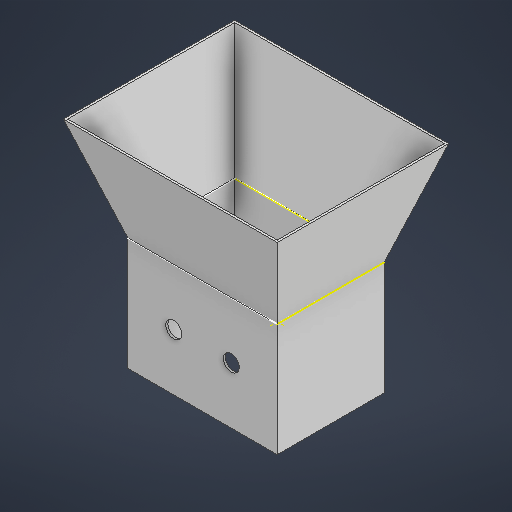
# Autodesk Inventor part: tolva
Saved by Autodesk Inventor 2026.1 (Build 301233020, 233B)
## iProperties
Created: 2025-11-30
Part Number: tolva
Material: Genérico
Document SubType Name: Modeling
Designer: TUF GAMING F15
Density: 1 g/cm^3
Appearance: Valor por defecto
Author: TUF GAMING F15
Autodesk Inventor part; units mm, degrees
ref_plane "YZ Plane" through (0, 0, 0) normal (1, 0, 0) x (0, 1, 0)
ref_plane "XZ Plane" through (0, 0, 0) normal (0, 1, 0) x (-1, 0, 0)
sketch "Boceto1" plane through (0, 0, 0) normal (0, 0, 1) x (1, 0, 0)
  circle A0 centre (0, 0) radius 62.5 construction
  circle A1 centre (0, 0) radius 20 construction
  line L0 (20, 0) -> (84, 0)
  circle A2 centre (84, 0) radius 62.5 construction
  circle A3 centre (84, 0) radius 20 construction
  line L1 (-62.5, 0) -> (-64, 0) construction
  line L2 (146.5, 0) -> (148, 0) construction
  line L3 (0, 62.5) -> (0, 82.5) construction
  line L4 (-64, 0) -> (-64, 82.5) construction
  line L5 (-64, 82.5) -> (0, 82.5)
  line L6 (0, 82.5) -> (148, 82.5)
  line L7 (148, 82.5) -> (148, 0) construction
  line L8 (-64, 0) -> (-64, -82.5) construction
  line L9 (-64, -82.5) -> (0, -82.5)
  line L10 (0, -82.5) -> (148, -82.5)
  line L11 (148, -82.5) -> (148, 0) construction
  line L12 (-64, 82.5) -> (-67, 82.5)
  line L13 (-67, 82.5) -> (-67, -82.5)
  line L14 (-67, -82.5) -> (-64, -82.5)
  line L15 (148, 82.5) -> (151, 82.5)
  line L16 (151, 82.5) -> (151, -82.5)
  line L17 (151, -82.5) -> (148, -82.5)
  circle A4 centre (0, 0) radius 12.7 construction
  line L18 (0, 12.7) -> (8.9803, 8.9803) construction
  line L19 (8.9803, 8.9803) -> (12.7, 0) construction
  line L20 (12.7, 0) -> (8.9803, -8.9803) construction
  line L21 (8.9803, -8.9803) -> (0, -12.7) construction
  line L22 (0, -12.7) -> (-8.9803, -8.9803) construction
  line L23 (-8.9803, -8.9803) -> (-12.7, 0) construction
  line L24 (-12.7, 0) -> (-8.9803, 8.9803) construction
  line L25 (-8.9803, 8.9803) -> (0, 12.7) construction
  circle A5 centre (0, 0) radius 11.7333
  circle A6 centre (84, 0) radius 12.7 construction
  line L26 (84, 12.7) -> (92.9803, 8.9803) construction
  line L27 (92.9803, 8.9803) -> (96.7, 0) construction
  line L28 (96.7, 0) -> (92.9803, -8.9803) construction
  line L29 (92.9803, -8.9803) -> (84, -12.7) construction
  line L30 (84, -12.7) -> (75.0197, -8.9803) construction
  line L31 (75.0197, -8.9803) -> (71.3, 0) construction
  line L32 (71.3, 0) -> (75.0197, 8.9803) construction
  line L33 (75.0197, 8.9803) -> (84, 12.7) construction
  circle A7 centre (84, 0) radius 11.7333
  dimension "d1" = 40
  dimension "d3" = 125
  dimension "d35" = 25.4
  dimension "d36" = 25.4
  dimension "d0" = 125
  dimension "d2" = 64
  dimension "d4" = 40
  dimension "d5" = 1.5
  dimension "d6" = 1.5
  dimension "d7" = 20
  dimension "d8" = 3
  dimension "d9" = 3
  constraints: 68 end point, 11 coincident, 6 perpendicular, 5 horizontal, 4 centre point, 3 symmetric about line, 2 horizontal alignment, 2 point on circle, 2 point on line, 2 vertical, 2 vertical alignment, 42 other
  measures "d0" diameter of A0
  measures "d2" distance of L0.start L0.end
  measures "d4" diameter of A3
  measures "d5" distance of L1.start L1.end
  measures "d6" distance of L2.start L2.end
  measures "d7" distance of L3.start L3.end
  measures "d8" distance of L4.end L12.end
  measures "d9" distance of L6.end L15.end
extrude "Extrusión1" add sketch "Boceto1" along normal blind 3
sketch "Boceto2" plane through (0, 0, 3) normal (0, 0, 1) x (1, 0, 0)
  line L0 (151, 82.5) -> (-67, 82.5) projected
  line L1 (-67, 82.5) -> (-64, 82.5)
  line L2 (-64, 82.5) -> (-64, -82.5)
  line L3 (-67, -82.5) -> (151, -82.5) projected
  line L4 (-67, 82.5) -> (-67, -82.5)
  line L5 (-64, -82.5) -> (-67, -82.5)
  line L6 (151, 82.5) -> (148, 82.5)
  line L7 (148, 82.5) -> (148, -82.5)
  line L8 (151, -82.5) -> (151, 82.5) projected
  line L9 (148, -82.5) -> (151, -82.5)
  line L10 (151, -82.5) -> (151, 82.5)
  point P0 (0, 0)
  dimension "d12" = 3
  dimension "d13" = 3
  constraints: 16 end point, 4 point on line, 3 perpendicular, 1 collinear, 1 horizontal, 1 vertical
  measures "d12" distance of L0.end L1.end
  measures "d13" distance of L0.start L6.end
extrude "Extrusión2" add sketch "Boceto2" along normal blind 75 contours L8 L3 L7 L0 | L2 L3 L4 L0
mirror "Simetría1" about plane through (149.5, 0, 78) normal (0, 0, 1) of "Extrusión2", "Extrusión1"
ref_plane "Plano de trabajo1" through (-67, 232.5, 0) normal (0, 1, 0) x (1, 0, 0)
sketch "Boceto4" plane through (-67, 232.5, 0) normal (0, 1, 0) x (1, 0, 0)
  line L0 (215, -153) -> (3, -153) projected
  line L1 (3, -153) -> (3, -203) construction
  line L2 (3, -153) -> (-47, -153) construction
  line L3 (3, -153) -> (53, -153) construction
  line L4 (215, -3) -> (215, -153) projected
  line L5 (215, -3) -> (215, 47) construction
  line L6 (215, -3) -> (265, -3) construction
  line L7 (215, -3) -> (265, -3) construction
  line L8 (265, -3) -> (265, 47) construction
  line L9 (265, 47) -> (215, 47) construction
  line L10 (3, -203) -> (-47, -203) construction
  line L11 (-47, -203) -> (-47, -153) construction
  line L12 (-47, -203) -> (265, -203)
  line L13 (265, -203) -> (265, 47)
  line L14 (265, 47) -> (-47, 47)
  line L15 (-47, 47) -> (-47, -203)
  line L16 (-47, -203) -> (-47, -206) construction
  line L17 (-47, -203) -> (-50, -203) construction
  line L18 (-50, -203) -> (-50, -206) construction
  line L19 (-50, -206) -> (-47, -206) construction
  line L20 (265, 47) -> (268, 47) construction
  line L21 (265, 47) -> (265, 50) construction
  line L22 (265, 50) -> (268, 50) construction
  line L23 (268, 50) -> (268, 47) construction
  line L24 (-50, -206) -> (268, -206)
  line L25 (268, -206) -> (268, 50)
  line L26 (268, 50) -> (-50, 50)
  line L27 (-50, 50) -> (-50, -206)
  point P0 (67, 0)
  dimension "d18" = 50
  dimension "d20" = 50
  dimension "d21" = 180
  dimension "d22" = 50
  dimension "d24" = 50
  dimension "d25" = 0
  dimension "d26" = 3
  dimension "d27" = 3
  dimension "d28" = 3
  dimension "d29" = 3
  constraints: 52 end point, 10 perpendicular, 7 horizontal, 5 parallel, 4 vertical, 2 collinear
  measures "d18" distance of L0.end L1.end
  measures "d20" distance of L0.end L2.end
  measures "d21" angle of L2 L3
  measures "d22" distance of L4.start L5.end
  measures "d24" distance of L4.start L6.end
  measures "d25" distance between parallel lines of L6 L7
  measures "d26" distance of L10.end L16.end
  measures "d27" distance of L10.end L17.end
  measures "d28" distance of L8.end L20.end
  measures "d29" distance of L8.end L21.end
sketch "Boceto5" plane through (-67, 82.5, 0) normal (0, 1, 0) x (1, 0, 0)
  line L0 (218, 0) -> (0, 0) projected
  line L1 (218, 0) -> (218, -156) projected
  line L2 (0, 0) -> (218, 0)
  line L3 (218, 0) -> (218, -156)
  line L4 (218, -156) -> (0, -156)
  line L5 (0, -156) -> (0, 0)
  line L6 (215, -3) -> (3, -3) projected
  line L7 (3, -3) -> (215, -3)
  line L8 (215, -3) -> (215, -153)
  line L9 (215, -153) -> (3, -153)
  line L10 (3, -153) -> (3, -3)
  point P0 (67, 0)
  constraints: 16 end point, 4 parallel, 2 horizontal, 2 perpendicular
loft "Solevación1" add profiles "Boceto4" section 1 edges at (151, 82.5, 78) (42, 82.5, 0) (-67, 82.5, 78) (42, 82.5, 156) contours L15 L14 L13 L12
shell "Vaciado1" thickness 3 removed faces 2 at (94, 232.5, 119.6667) at (77.3333, 82.5, 103)
